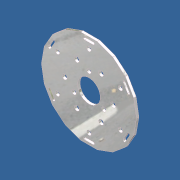
# Autodesk Inventor part: Traction Wheel Side Plate 1764
Saved by Autodesk Inventor 2011 (Build 150239000, 239)
## iProperties
Created: 2010-01-10
Part Number: Traction Wheel Side Plate 1764
Document SubType Name: Modeling
Designer: wbridges
Density: 1 g/cm^3
Author: wbridges
Autodesk Inventor part; units mm, degrees
ref_plane "YZ Plane" through (0, 0, 0) normal (1, 0, 0) x (0, 1, 0)
ref_plane "XZ Plane" through (0, 0, 0) normal (0, 1, 0) x (-1, 0, 0)
ref_plane "XY Plane" through (0, 0, 0) normal (0, 0, 1) x (1, 0, 0)
sketch "Sketch1" plane through (0, 0, 0) normal (0, 0, 1) x (1, 0, 0)
  arc A0 (4.2545, 41.275) -> (4.2545, 43.688) centre (4.2545, 42.4815) ccw
  line L0 (4.2545, 41.275) -> (-4.2545, 41.275)
  arc A1 (-4.2545, 43.688) -> (-4.2545, 41.275) centre (-4.2545, 42.4815) ccw
  line L1 (-4.2545, 43.688) -> (4.2545, 43.688)
  circle A2 centre (0, 35.660965) radius 2.16535
  circle A3 centre (0, 16.8275) radius 2.16535
  circle A4 centre (11.93165, 20.666224) radius 2.4384
  circle A5 centre (0, 0) radius 11.1125
  circle A6 centre (0, 0) radius 21.4249
  circle A7 centre (-11.93165, 20.666224) radius 2.4384
  circle A8 centre (-23.8633, 0) radius 2.4384
  circle A9 centre (-11.93165, -20.666224) radius 2.4384
  circle A10 centre (11.93165, -20.666224) radius 2.4384
  circle A11 centre (23.8633, 0) radius 2.4384
  line L2 (-11.93165, 20.666224) -> (11.93165, 20.666224)
  circle A12 centre (-14.573042, -8.41375) radius 2.16535
  circle A13 centre (14.573042, -8.41375) radius 2.16535
  arc A14 (-33.617949, 24.322005) -> (-35.707668, 25.528505) centre (-34.662808, 24.925255) ccw
  arc A15 (-39.962168, 18.159495) -> (-37.872449, 16.952995) centre (-38.917308, 17.556245) ccw
  line L3 (-39.962168, 18.159495) -> (-35.707668, 25.528505)
  line L4 (-33.617949, 24.322005) -> (-37.872449, 16.952995)
  circle A16 centre (-30.883302, 17.830483) radius 2.16535
  circle A17 centre (-23.8633, 0) radius 2.4384
  arc A18 (-37.872449, -16.952995) -> (-39.962168, -18.159495) centre (-38.917308, -17.556245) ccw
  arc A19 (-35.707668, -25.528505) -> (-33.617949, -24.322005) centre (-34.662808, -24.925255) ccw
  line L5 (-35.707668, -25.528505) -> (-39.962168, -18.159495)
  line L6 (-37.872449, -16.952995) -> (-33.617949, -24.322005)
  circle A20 centre (-30.883302, -17.830482) radius 2.16535
  circle A21 centre (-11.93165, -20.666224) radius 2.4384
  arc A22 (-4.2545, -41.275) -> (-4.2545, -43.688) centre (-4.2545, -42.4815) ccw
  arc A23 (4.2545, -43.688) -> (4.2545, -41.275) centre (4.2545, -42.4815) ccw
  line L7 (4.2545, -43.688) -> (-4.2545, -43.688)
  line L8 (-4.2545, -41.275) -> (4.2545, -41.275)
  circle A24 centre (0, -35.660965) radius 2.16535
  circle A25 centre (11.93165, -20.666224) radius 2.4384
  arc A26 (33.617949, -24.322005) -> (35.707668, -25.528505) centre (34.662808, -24.925255) ccw
  arc A27 (39.962168, -18.159495) -> (37.872449, -16.952995) centre (38.917308, -17.556245) ccw
  line L9 (39.962168, -18.159495) -> (35.707668, -25.528505)
  line L10 (33.617949, -24.322005) -> (37.872449, -16.952995)
  circle A28 centre (30.883302, -17.830483) radius 2.16535
  circle A29 centre (23.8633, 0) radius 2.4384
  arc A30 (37.872449, 16.952995) -> (39.962168, 18.159495) centre (38.917308, 17.556245) ccw
  arc A31 (35.707668, 25.528505) -> (33.617949, 24.322005) centre (34.662808, 24.925255) ccw
  line L11 (35.707668, 25.528505) -> (39.962168, 18.159495)
  line L12 (37.872449, 16.952995) -> (33.617949, 24.322005)
  circle A32 centre (30.883302, 17.830482) radius 2.16535
  circle A33 centre (11.93165, 20.666224) radius 2.4384
  line L13 (-46.747703, 0) -> (-43.928471, 15.988656)
  line L14 (-43.928471, 15.988656) -> (-35.810818, 30.048844)
  line L15 (-35.810818, 30.048844) -> (-23.373851, 40.484698)
  line L16 (-23.373851, 40.484698) -> (-8.117653, 46.0375)
  line L17 (-8.117653, 46.0375) -> (8.117653, 46.0375)
  line L18 (8.117653, 46.0375) -> (23.373851, 40.484698)
  line L19 (23.373851, 40.484698) -> (35.810818, 30.048844)
  line L20 (35.810818, 30.048844) -> (43.928471, 15.988656)
  line L21 (43.928471, 15.988656) -> (46.747703, 0)
  line L22 (46.747703, 0) -> (43.928471, -15.988656)
  line L23 (43.928471, -15.988656) -> (35.810818, -30.048844)
  line L24 (35.810818, -30.048844) -> (23.373851, -40.484698)
  line L25 (23.373851, -40.484698) -> (8.117653, -46.0375)
  line L26 (8.117653, -46.0375) -> (-8.117653, -46.0375)
  line L27 (-8.117653, -46.0375) -> (-23.373851, -40.484698)
  line L28 (-23.373851, -40.484698) -> (-35.810818, -30.048844)
  line L29 (-35.810818, -30.048844) -> (-43.928471, -15.988656)
  line L30 (-43.928471, -15.988656) -> (-46.747703, 0)
  line L31 (-4.2545, 43.688) -> (-4.2545, 41.275)
  point P0 (0, 41.275)
  point P1 (0, 43.688)
  point P2 (-35.745199, 20.6375)
  point P3 (-37.834918, 21.844)
  point P4 (-35.745199, -20.6375)
  point P5 (-37.834918, -21.844)
  point P6 (0, -41.275)
  point P7 (0, -43.688)
  point P8 (35.745199, -20.6375)
  point P9 (37.834918, -21.844)
  point P10 (35.745199, 20.6375)
  point P11 (37.834918, 21.844)
  point P12 (0, 46.0375)
  dimension "d1" = 2.413
  dimension "d2" = 8.509
  dimension "d7" = 4.3307
  dimension "d9" = 4.8768
  dimension "d11" = 5.61404
  dimension "d13" = 16.8275
  dimension "d14" = 22.225
  dimension "d16" = 42.8498
  dimension "d19" = 360
  dimension "d25" = 360
  dimension "d29" = 360
  dimension "d33" = 92.075
  dimension "d35" = 8.509
  dimension "d36" = 82.55
  constraints: 64 end point, 34 centre point, 25 point on circle, 5 vertical alignment, 4 coincident, 4 midpoint, 3 parallel, 1 equal radius, 1 horizontal, 1 perpendicular, 1 tangent, 154 other
  measures "d1" distance between parallel lines of L1 L0
  measures "d2" distance of L0.start L0.end
  measures "d7" diameter of A2
  measures "d9" diameter of A4
  measures "d11" distance of A2.centre point (0, 41.275)
  measures "d13" distance of point (0, 0) A3.centre
  measures "d14" diameter of A5
  measures "d16" diameter of A6
  measures "d33" distance between parallel lines of L22 L13
  measures "d35" distance of A0.centre A1.centre
  measures "d36" distance between parallel lines of L8 L0
extrude "Extrusion1" add sketch "Sketch1" along normal blind 2.413 contours A4 A6 L2 | A6 L2 | L2 A6 | A6 A7 L2 | L13 L14 L15 L16 L17 L18 L19 L20 L21 L22 L23 L24 L25 L26 L27 L28 L29 L30
body "Solid1"
